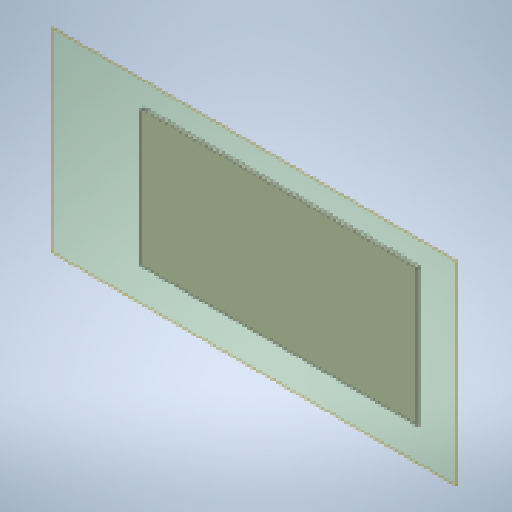
# Autodesk Inventor part: acrylicDoor
Saved by Autodesk Inventor 2024.3 (Build 283343000, 343)
## iProperties
Created: 2025-06-11
Part Number: acrylicDoor
Material: Generic
Document SubType Name: Modeling
Designer: megha
Density: 1 g/cm^3
Appearance: Default
Author: megha
Autodesk Inventor part; units mm, degrees
ref_plane "YZ Plane" through (0, 0, 0) normal (1, 0, 0) x (0, 1, 0)
ref_plane "XZ Plane" through (0, 0, 0) normal (0, 1, 0) x (-1, 0, 0)
ref_plane "XY Plane" through (0, 0, 0) normal (0, 0, 1) x (1, 0, 0)
ref_plane "Work Plane1" through (98.003, 24.491, 144.9473) normal (0, -0.0001, -1) x (0, -1, 0.0001)
sketch "Sketch1" plane through (98.003, 24.491, 144.9473) normal (0, -0.0001, -1) x (0, -1, 0.0001)
  line L0 (3.4596, -1.4381) -> (98.1832, -4.2342) projected
  arc A0 (-4.7625, 4.7625) -> (3.4596, -1.4381) centre (0, 4.7625) ccw projected
  line L1 (3.4596, 0) -> (98.1832, 0) projected
  line L2 (94.7649, -4.2342) -> (94.7649, 8) projected
  line L3 (94.7649, 8) -> (81.7675, 8) projected
  line L4 (81.7675, 8) -> (81.7675, 170.35)
  line L5 (81.7675, 170.35) -> (94.7649, 170.35) projected
  line L6 (94.7649, 170.35) -> (94.7649, 178.35) projected
  arc A1 (0, 178.35) -> (-4.7625, 173.5875) centre (0, 173.5875) ccw
  line L7 (78.7675, 8) -> (0.2375, 8)
  line L8 (0.2375, 8) -> (-4.7625, 8)
  line L9 (78.7675, 8) -> (81.7675, 8)
  line L10 (81.7675, 170.35) -> (81.7675, 178.35)
  line L11 (0, 178.35) -> (81.7675, 178.35)
  line L12 (-4.7625, 8) -> (-4.7625, 173.5875)
  line L13 (-2.7625, 173.5875) -> (-2.7625, 10)
  line L14 (79.7675, 10) -> (79.7675, 170.35)
  line L15 (79.7675, 170.35) -> (79.7675, 176.35)
  line L16 (79.7675, 176.35) -> (0, 176.35)
  arc A2 (0, 176.35) -> (-2.7625, 173.5875) centre (0, 173.5875) ccw
  line L17 (-2.7625, 10) -> (-2.7625, 8)
  line L18 (79.7675, 10) -> (79.7675, 8)
  point P0 (24.483, 98.003)
  dimension "d2" = 2
  constraints: 26 end point, 5 point on circle, 2 centre point, 2 perpendicular, 2 point on line, 1 collinear, 1 horizontal, 1 vertical, 4 other
  measures "d2" distance between parallel lines of L12 L13
extrude "Extrusion1" add sketch "Sketch1" along normal blind 1.5875 contours L9 L7 L8 L17 L13 A2 L16 L15 L14 L18
sketch "Sketch2" plane through (98.003, 24.4909, 143.3598) normal (0, -0.0001, -1) x (-1, 0, 0)
  circle A0 centre (10.4064, -19.902) radius 0.625
  circle A1 centre (10.4064, -26.152) radius 0.625
  point P0 (98.003, -24.483)
  constraints: 2 centre point
extrude "Extrusion2" cut sketch "Sketch2" against normal blind 1.5875
body "Solid1"
